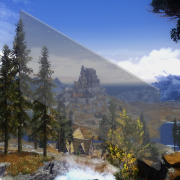
# Autodesk Inventor part: C16_TK_ElectricBoard
Saved by Autodesk Inventor 2015 SP1 (Build 190203100, 203)
## iProperties
Created: 2016-01-21
Part Number: C16_TK_ElectricBoard
Material: Polycarbonate, Clear
Document SubType Name: Modeling
Designer: TheeTimatahee
Density: 1.2 g/cm^3
Appearance: Polycarbonate - Clear
Mass: 531.119 g
Surface Area: 1933.13 cm^2
Volume: 442.599 cm^3
Author: TheeTimatahee
Autodesk Inventor part; units mm, degrees
ref_plane "YZ Plane" through (0, 0, 0) normal (1, 0, 0) x (0, 1, 0)
ref_plane "XZ Plane" through (0, 0, 0) normal (0, 1, 0) x (-1, 0, 0)
ref_plane "XY Plane" through (0, 0, 0) normal (0, 0, 1) x (1, 0, 0)
sketch "Sketch1" plane through (0, 0, 0) normal (0, 0, 1) x (1, 0, 0)
  line L0 (-215.9, -107.95) -> (215.9, -107.95)
  line L1 (215.9, -107.95) -> (215.9, 107.95)
  line L2 (215.9, 107.95) -> (-215.9, 107.95)
  line L3 (-215.9, 107.95) -> (-215.9, -107.95)
  line L4 (-215.9, -107.95) -> (215.9, 107.95) construction
  line L5 (215.9, -107.95) -> (-215.9, 107.95) construction
  point P0 (0, 0)
  dimension "d0" = 215.9
  dimension "d1" = 431.8
  constraints: 12 end point, 2 midpoint, 2 parallel, 1 horizontal, 1 perpendicular
  measures "d0" distance of L0.end L1.end
  measures "d1" distance of L1.end L2.end
extrude "Extrusion1" add sketch "Sketch1" along normal blind 4.7625
sketch "Sketch2" plane through (0, 0, 4.7625) normal (0, 0, 1) x (1, 0, 0)
  line L0 (215.9, -107.95) -> (215.9, 107.95) projected
  line L1 (215.9, 107.95) -> (-215.9, 107.95) projected
  line L2 (-215.9, -107.95) -> (215.9, -107.95) projected
  point P0 (0, 0)
  point P1 (127, 95.25)
  point P2 (190.5, -95.25)
  point P3 (101.6, 95.25)
  point P4 (76.2, 95.25)
  point P5 (50.8, 95.25)
  point P6 (25.4, 95.25)
  point P7 (0, 95.25)
  point P8 (-25.4, 95.25)
  point P9 (-50.8, 95.25)
  point P10 (-76.2, 95.25)
  point P11 (-101.6, 95.25)
  point P12 (-127, 95.25)
  point P13 (139.7, -95.25)
  point P14 (88.9, -95.25)
  point P15 (38.1, -95.25)
  point P16 (-12.7, -95.25)
  point P17 (12.7, -95.25)
  point P18 (-38.1, -95.25)
  point P19 (-88.9, -95.25)
  point P20 (-139.7, -95.25)
  point P21 (-190.5, -95.25)
  dimension "d12" = 88.9
  dimension "d13" = 12.7
  dimension "d14" = 25.4
  dimension "d15" = 12.7
  dimension "d18" = 25.4
  dimension "d25" = 50.8
  dimension "d30" = 25.4
  dimension "d31" = 12.7
  dimension "d32" = 25.4
  dimension "d33" = 12.7
  dimension "d36" = 50.8
  constraints: 3 horizontal, 17 other
  measures "d12" distance from line of L0 point (127, 95.25)
  measures "d13" distance from line of L1 point (127, 95.25)
  measures "d14" distance from line of L0 point (190.5, -95.25)
  measures "d15" distance from line of L2 point (190.5, -95.25)
  measures "d18" distance of point (127, 95.25) point (101.6, 95.25)
  measures "d25" distance of point (190.5, -95.25) point (139.7, -95.25)
  measures "d30" distance of point (38.1, -95.25) point (12.7, -95.25)
  measures "d31" distance from line of L2 point (12.7, -95.25)
  measures "d32" distance of point (-12.7, -95.25) point (-38.1, -95.25)
  measures "d33" distance from line of L2 point (-38.1, -95.25)
  measures "d36" distance of point (-38.1, -95.25) point (-88.9, -95.25)
hole "Hole1" at (127, 95.25, 4.7625) at (101.6, 95.25, 4.7625) at (76.2, 95.25, 4.7625) at (50.8, 95.25, 4.7625) at (25.4, 95.25, 4.7625) at (0, 95.25, 4.7625) at (-25.4, 95.25, 4.7625) at (-50.8, 95.25, 4.7625) at (-76.2, 95.25, 4.7625) at (-101.6, 95.25, 4.7625) at (-127, 95.25, 4.7625) at (190.5, -95.25, 4.7625) at (139.7, -95.25, 4.7625) at (88.9, -95.25, 4.7625) at (38.1, -95.25, 4.7625) at (12.7, -95.25, 4.7625) at (-12.7, -95.25, 4.7625) at (-38.1, -95.25, 4.7625) at (-88.9, -95.25, 4.7625) at (-139.7, -95.25, 4.7625) at (-190.5, -95.25, 4.7625) direction (0, 0, -1) diameter 4.1402 end through all
fillet "Fillet1" radius 3.175 4 edges at (215.9, -107.95, 2.3813) (-215.9, -107.95, 2.3813) (-215.9, 107.95, 2.3813) (215.9, 107.95, 2.3813)
body "Solid1"
